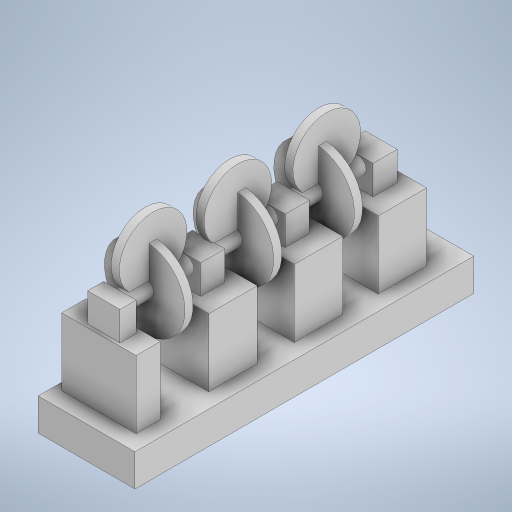
# Autodesk Inventor part: Pieza1
Saved by Autodesk Inventor 2024 (Build 280153000, 153)
## iProperties
Created: 2024-01-29
Part Number: Pieza1
Material: Genérico
Document SubType Name: Modeling
Designer: DANIELA GALEANO
Density: 1 g/cm^3
Appearance: Valor por defecto
Author: DANIELA GALEANO
Autodesk Inventor part; units mm, degrees
ref_plane "YZ Plane" through (0, 0, 0) normal (1, 0, 0) x (0, 1, 0)
ref_plane "XZ Plane" through (0, 0, 0) normal (0, 1, 0) x (-1, 0, 0)
ref_plane "XY Plane" through (0, 0, 0) normal (0, 0, 1) x (1, 0, 0)
sketch "Boceto1" plane through (0, 0, 0) normal (0, 1, 0) x (-1, 0, 0)
  line L0 (43.6381, 98.6893) -> (-16.3619, 98.6893)
  line L1 (-16.3619, 98.6893) -> (-16.3619, -111.3107)
  line L2 (-16.3619, -111.3107) -> (43.6381, -111.3107)
  line L3 (43.6381, -111.3107) -> (43.6381, 98.6893)
  point P0 (0, 0)
  dimension "d0" = 210
  dimension "d1" = 60
  constraints: 8 end point, 2 parallel, 1 horizontal, 1 perpendicular
  measures "d0" distance of L2.end L0.start
  measures "d1" distance of L1.end L2.end
extrude "Extrusión1" add sketch "Boceto1" along normal blind 20
sketch "Boceto2" plane through (0, 20, 0) normal (0, 1, 0) x (1, 0, 0)
  line L0 (-38.9219, -88.6893) -> (7.0781, -88.6893)
  line L1 (7.0781, -88.6893) -> (7.0781, -73.6893)
  line L2 (7.0781, -73.6893) -> (-38.9219, -73.6893)
  line L3 (-38.9219, -73.6893) -> (-38.9219, -88.6893)
  line L4 (-38.9219, -43.6893) -> (7.0781, -43.6893)
  line L5 (7.0781, -43.6893) -> (7.0781, -13.6893)
  line L6 (7.0781, -13.6893) -> (-38.9219, -13.6893)
  line L7 (-38.9219, -13.6893) -> (-38.9219, -43.6893)
  line L8 (-38.9219, 9.3107) -> (7.0781, 9.3107)
  line L9 (7.0781, 9.3107) -> (7.0781, 39.3107)
  line L10 (7.0781, 39.3107) -> (-38.9219, 39.3107)
  line L11 (-38.9219, 39.3107) -> (-38.9219, 9.3107)
  line L12 (-38.9219, 61.3107) -> (7.0781, 61.3107)
  line L13 (7.0781, 61.3107) -> (7.0781, 91.3107)
  line L14 (7.0781, 91.3107) -> (-38.9219, 91.3107)
  line L15 (-38.9219, 91.3107) -> (-38.9219, 61.3107)
  line L16 (-43.6381, -98.6893) -> (16.3619, -98.6893) projected
  line L17 (16.3619, 111.3107) -> (-43.6381, 111.3107) projected
  point P0 (0, 0)
  dimension "d6" = 15
  dimension "d7" = 30
  dimension "d8" = 46
  dimension "d9" = 46
  dimension "d10" = 30
  dimension "d11" = 46
  dimension "d12" = 30
  dimension "d13" = 46
  dimension "d14" = 10
  dimension "d15" = 20
  dimension "d16" = 30
  dimension "d17" = 23
  dimension "d18" = 22
  constraints: 32 end point, 8 parallel, 4 horizontal, 4 perpendicular, 3 point on line
  measures "d6" distance of L0.end L1.end
  measures "d7" distance of L6.end L4.start
  measures "d8" distance of L4.start L4.end
  measures "d9" distance of L9.end L10.end
  measures "d10" distance of L10.end L8.start
  measures "d11" distance of L13.end L14.end
  measures "d12" distance of L14.end L12.start
  measures "d13" distance of L0.start L0.end
  measures "d14" distance between parallel lines of L16 L0
  measures "d15" distance between parallel lines of L17 L14
  measures "d16" distance between parallel lines of L2 L4
  measures "d17" distance between parallel lines of L6 L8
  measures "d18" distance between parallel lines of L10 L12
extrude "Extrusión2" add sketch "Boceto2" along normal blind 42
sketch "Boceto3" plane through (0, 62, 0) normal (0, 1, 0) x (1, 0, 0)
  line L0 (-4.7048, -21.9668) -> (-24.7048, -21.9668)
  line L1 (-24.7048, -21.9668) -> (-24.7048, -36.9668)
  line L2 (-24.7048, -36.9668) -> (-4.7048, -36.9668)
  line L3 (-4.7048, -36.9668) -> (-4.7048, -21.9668)
  line L4 (-24.7048, 15.3623) -> (-4.7048, 15.3623)
  line L5 (-4.7048, 15.3623) -> (-4.7048, 30.3623)
  line L6 (-4.7048, 30.3623) -> (-24.7048, 30.3623)
  line L7 (-24.7048, 30.3623) -> (-24.7048, 15.3623)
  line L8 (-24.7048, 69.8642) -> (-4.7048, 69.8642)
  line L9 (-4.7048, 69.8642) -> (-4.7048, 84.8642)
  line L10 (-4.7048, 84.8642) -> (-24.7048, 84.8642)
  line L11 (-24.7048, 84.8642) -> (-24.7048, 69.8642)
  line L12 (-24.7048, -86.9407) -> (-4.7048, -86.9407)
  line L13 (-4.7048, -86.9407) -> (-4.7048, -76.9407)
  line L14 (-4.7048, -76.9407) -> (-24.7048, -76.9407)
  line L15 (-24.7048, -76.9407) -> (-24.7048, -86.9407)
  point P0 (0, 0)
  dimension "d19" = 20
  dimension "d20" = 15
  dimension "d21" = 20
  dimension "d22" = 15
  dimension "d23" = 15
  dimension "d24" = 20
  dimension "d25" = 20
  dimension "d26" = 10
  dimension "d31" = 0
  constraints: 32 end point, 8 parallel, 4 horizontal, 4 perpendicular, 4 point on line
  measures "d19" distance of L0.start L0.end
  measures "d20" distance of L0.end L1.end
  measures "d21" distance of L4.start L4.end
  measures "d22" distance of L6.end L4.start
  measures "d23" distance of L10.end L8.start
  measures "d24" distance of L8.start L8.end
  measures "d25" distance of L13.end L14.end
  measures "d26" distance of L14.end L12.start
  measures "d31" distance between parallel lines of L13 L3
extrude "Extrusión3" add sketch "Boceto3" along normal blind 18
sketch "Boceto4" plane through (-4.7048, 62, -84.8642) normal (0, 0, -1) x (-1, 0, 0)
  circle A0 centre (9.6513, 12.486) radius 5.5025
  point P0 (-4.7048, -62)
  constraints: 1 centre point
extrude "Extrusión4" add sketch "Boceto4" against normal blind 170
ref_plane "Plano de trabajo1" through (-24.7048, 62, 56.9407) normal (0, 0, 1) x (1, 0, 0)
sketch "Boceto6" plane through (-24.7048, 62, 56.9407) normal (0, 0, 1) x (1, 0, 0)
  circle A0 centre (10.3487, 12.486) radius 5.5025 projected
  circle A1 centre (10.3487, 12.486) radius 25
  point P0 (24.7048, -62)
  point P1 (41.0667, -62)
  dimension "d33" = 74.486
  dimension "d34" = 25
  constraints: 1 centre point, 1 coincident
  measures "d33" vertical distance of point (41.067, -62) A1.centre
  measures "d34" radius of A1
extrude "Extrusión5" add sketch "Boceto6" along normal blind 5 contours A0 | A1
ref_plane "Plano de trabajo3" through (-24.7048, 62, 1.9407) normal (0, 0, 1) x (1, 0, 0)
ref_plane "Plano de trabajo4" through (-24.7048, 62, -48.0593) normal (0, 0, 1) x (1, 0, 0)
sketch "Boceto7" plane through (-24.7048, 62, 1.9407) normal (0, 0, 1) x (1, 0, 0)
  circle A0 centre (10.3487, 12.486) radius 25 projected
  circle A1 centre (10.3487, 12.486) radius 20
  point P0 (24.7048, -62)
  constraints: 1 centre point, 1 coincident
extrude "Extrusión6" add sketch "Boceto7" along normal blind 5 contours A0 | A1
sketch "Boceto8" plane through (-24.7048, 62, -48.0593) normal (0, 0, 1) x (1, 0, 0)
  circle A0 centre (10.3487, 12.486) radius 25 projected
  circle A1 centre (10.3487, 12.486) radius 20
  point P0 (24.7048, -62)
  dimension "d48" = 50
  constraints: 1 centre point, 1 coincident
  measures "d48" diameter of A0
extrude "Extrusión7" add sketch "Boceto8" along normal blind 5 contours A0 | A1
ref_plane "Plano de trabajo5" through (-14.3562, 74.486, 59.4407) normal (0, 0, -1) x (-1, 0, 0)
sketch "Boceto10" plane through (-14.3562, 74.486, 59.4407) normal (0, 0, -1) x (-1, 0, 0)
  line L0 (-2.688, 19.6173) -> (2.312, 19.6173)
  line L1 (2.312, 19.6173) -> (2.312, -1.3827)
  line L2 (2.312, -1.3827) -> (-2.688, -1.3827)
  line L3 (-2.688, -1.3827) -> (-2.688, 19.6173)
  line L4 (-30.7181, -74.486) -> (29.2819, -74.486) projected
  point P0 (-14.3562, -74.486)
  dimension "d43" = 21
  dimension "d46" = 5
  constraints: 8 end point, 2 parallel, 1 horizontal, 1 perpendicular
  measures "d43" distance of L2.end L0.start
  measures "d46" distance of L0.start L0.end
revolve "Revolución1" add sketch "Boceto10" angle 360 about axis through (-11.6681, 94.1034, 59.4407) along (-1, 0, 0)
sketch "Boceto11" plane through (-14.3562, 74.486, 59.4407) normal (0, 0, -1) x (-1, 0, 0)
  point P0 (-14.3562, -74.486)
ref_plane "Plano de trabajo6" through (-22.9219, 20, 88.6893) normal (1, 0, 0) x (0, 0, -1)
sketch "Boceto14" plane through (-13.6381, 102.3503, 6.9407) normal (0, 0, 1) x (1, 0, 0)
  line L0 (-3.0387, -8.6715) -> (1.9613, -8.6715)
  line L1 (1.9613, -8.6715) -> (1.9613, -29.6715)
  line L2 (1.9613, -29.6715) -> (-3.0387, -29.6715)
  line L3 (-3.0387, -29.6715) -> (-3.0387, -8.6715)
  line L4 (-30.7181, -74.486) -> (29.2819, -74.486)
  point P0 (-14.3562, -74.486)
  dimension "d51" = 21
  dimension "d52" = 5
  constraints: 10 end point, 2 parallel, 1 horizontal, 1 perpendicular
  measures "d51" distance of L2.end L0.start
  measures "d52" distance of L0.start L0.end
revolve "Revolución2" add sketch "Boceto14" angle 360 about axis through (-16.6768, 93.6788, 6.9407) along (-1, 0, 0)
sketch "Boceto15" plane through (-23.9868, 103.3042, -48.0593) normal (0, 0, 1) x (1, 0, 0)
  line L0 (7.4215, -9.5056) -> (12.4215, -9.5056)
  line L1 (12.4215, -9.5056) -> (12.4215, -30.5056)
  line L2 (12.4215, -30.5056) -> (7.4215, -30.5056)
  line L3 (7.4215, -30.5056) -> (7.4215, -9.5056)
  line L4 (-30.7181, -74.486) -> (29.2819, -74.486)
  point P0 (-14.3562, -74.486)
  dimension "d54" = 21
  dimension "d55" = 5
  constraints: 10 end point, 2 parallel, 1 horizontal, 1 perpendicular
  measures "d54" distance of L2.end L0.start
  measures "d55" distance of L0.start L0.end
revolve "Revolución3" add sketch "Boceto15" angle 360 about axis through (-16.5652, 93.7986, -48.0593) along (-1, 0, 0)
